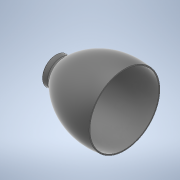
# Autodesk Inventor part: Screen
Saved by Autodesk Inventor 2020.2 (Build 242310000, 310)
## iProperties
Created: 2021-06-30
Part Number: Screen
Material: Generic
Document SubType Name: Modeling
Designer: JK
Density: 1 g/cm^3
Appearance: Smooth - Black
Author: JK
Autodesk Inventor part; units mm, degrees
ref_plane "YZ Plane" through (0, 0, 0) normal (1, 0, 0) x (0, 1, 0)
ref_plane "XZ Plane" through (0, 0, 0) normal (0, 1, 0) x (-1, 0, 0)
ref_plane "XY Plane" through (0, 0, 0) normal (0, 0, 1) x (1, 0, 0)
sketch "Sketch1" plane through (0, 0, 0) normal (0, 1, 0) x (-1, 0, 0)
  line L0 (1.8334, 0) -> (1.8334, 20)
  line L1 (-88.1666, 51.6) -> (-88.1666, 50)
  line L2 (-1.1666, 20.905) -> (-1.1666, 0)
  line L3 (-1.1666, 0) -> (1.8334, 0)
  arc A0 (-1.1666, 20.905) -> (-88.1666, 50) centre (-72.2845, -47.1307) ccw
  arc A1 (1.8334, 20) -> (-88.1666, 51.6) centre (-72.2845, -47.1307) ccw
  point P0 (0, 0)
  point P1 (-1.1666, 10.4525)
  dimension "d0" = 3
  dimension "d2" = 1.6
  dimension "d3" = 20
  dimension "d4" = 90
  dimension "d5" = 50
  dimension "d10" = 100
  constraints: 8 end point, 4 point on circle, 3 vertical, 2 centre point, 1 concentric, 1 horizontal alignment, 1 midpoint, 1 perpendicular
  measures "d0" distance between parallel lines of L0 L2
  measures "d2" distance of L1.end L1.start
  measures "d3" distance of L0.start L0.end
  measures "d4" horizontal distance of L0.end L1.end
  measures "d5" vertical distance of point (0, 0) L1.end
  measures "d10" radius of A1
revolve "Revolution1" add sketch "Sketch1" angle 360 about axis through (1.1666, 0, 0) along (-1, 0, 0)
sketch "Sketch2" plane through (1.1666, 0, 0) normal (1, 0, 0) x (0, 0, -1)
  circle A0 centre (0, 0) radius 13.875
  point P0 (0, 0)
  dimension "d7" = 27.75
  constraints: 1 centre point, 1 coincident
  measures "d7" diameter of A0
extrude "Extrusion1" cut sketch "Sketch2" against normal through all
sketch "Sketch3" plane through (-1.8334, 0, 0) normal (-1, 0, 0) x (0, 0, 1)
  circle A0 centre (0, 0) radius 13.875 projected
  circle A1 centre (0, 0) radius 20 projected
  point P0 (0, 0)
extrude "Extrusion2" add sketch "Sketch3" along normal blind 10
fillet "Fillet1" radius 5 1 edges at (-1.8334, 0, -20)
fillet "Fillet2" radius 1 1 edges at (-11.8334, 0, -20)
body "Solid1"
